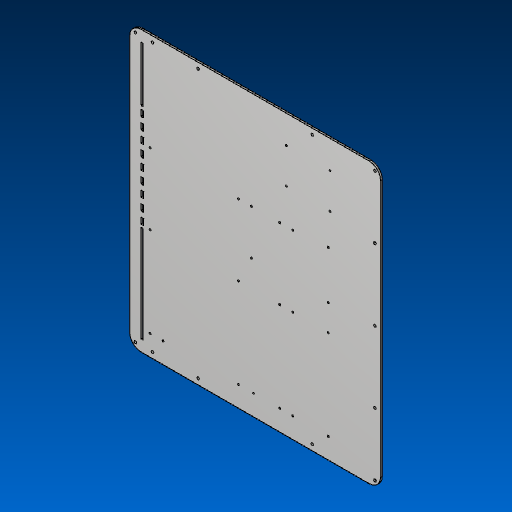
# Autodesk Inventor part: right_panel
Saved by Autodesk Inventor 2018 (Build 220112000, 112)
## iProperties
Created: 2019-10-14
Part Number: right_panel
Material: アルミニウム 6061
Document SubType Name: Modeling
Designer: gisen
Density: 2.7 g/cm^3
Appearance: アルミニウム - フラット
Author: gisen
Autodesk Inventor part; units mm, degrees
ref_plane "YZ Plane" through (0, 0, 0) normal (1, 0, 0) x (0, 1, 0)
ref_plane "XZ Plane" through (0, 0, 0) normal (0, 1, 0) x (-1, 0, 0)
ref_plane "XY Plane" through (0, 0, 0) normal (0, 0, 1) x (1, 0, 0)
sketch "スケッチ1" plane through (0, 0, 0) normal (0, 0, 1) x (1, 0, 0)
  line L0 (-200, -245) -> (200, -245)
  line L1 (220, -225) -> (220, 225)
  line L2 (200, 245) -> (-200, 245)
  line L3 (-220, 225) -> (-220, -225)
  line L4 (-220, -245) -> (220, 245) construction
  line L5 (220, -245) -> (-220, 245) construction
  circle A0 centre (-210, 235) radius 2.25
  circle A1 centre (210, 235) radius 2.25
  circle A2 centre (-210, -235) radius 2.25
  circle A3 centre (210, -235) radius 2.25
  arc A4 (-200, 245) -> (-220, 225) centre (-200, 225) ccw
  arc A5 (220, 225) -> (200, 245) centre (200, 225) ccw
  arc A6 (200, -245) -> (220, -225) centre (200, -225) ccw
  arc A7 (-220, -225) -> (-200, -245) centre (-200, -225) ccw
  point P0 (0, 0)
  dimension "d0" = 440
  dimension "d1" = 490
  dimension "d2" = 4.5
  dimension "d3" = 10
  dimension "d4" = 10
  dimension "d5" = 10
  dimension "d6" = 10
  dimension "d7" = 10
  dimension "d8" = 10
  dimension "d9" = 10
  dimension "d10" = 10
  dimension "d11" = 20
  constraints: 12 end point, 8 centre point, 8 point on circle, 8 point on line, 8 tangent, 6 equal radius, 2 midpoint, 2 parallel, 1 horizontal, 1 perpendicular
  measures "d0" distance of L5.end L4.end
  measures "d1" distance of L4.end L5.start
  measures "d2" diameter of A0
  measures "d3" distance from line of A0.centre L2
  measures "d4" distance from line of L3 A0.centre
  measures "d5" distance from line of A1.centre L2
  measures "d6" distance from line of L1 A1.centre
  measures "d7" distance from line of L1 A3.centre
  measures "d8" distance from line of L0 A3.centre
  measures "d9" distance from line of L0 A2.centre
  measures "d10" distance from line of L3 A2.centre
  measures "d11" radius of A4
extrude "押し出し1" add sketch "スケッチ1" along normal blind 3
sketch "スケッチ2" plane through (0, 0, 3) normal (0, 0, 1) x (1, 0, 0)
  circle A0 centre (43.092, 72.9258) radius 1.6
  circle A1 centre (-29.298, 72.9258) radius 1.6
  circle A2 centre (-184.238, 72.9258) radius 1.6
  circle A3 centre (-184.238, -51.5342) radius 1.6
  circle A4 centre (-161.378, -209.0142) radius 1.6
  circle A5 centre (-29.298, -209.0142) radius 1.6
  circle A6 centre (43.092, -209.0142) radius 1.6
  circle A7 centre (43.092, -51.5342) radius 1.6
  circle A8 centre (-29.298, -51.5342) radius 1.6
  circle A9 centre (43.092, -209.0142) radius 2.25 projected
  circle A10 centre (-161.378, -209.0142) radius 2.25 projected
  circle A11 centre (43.092, -51.5342) radius 2.25 projected
  circle A12 centre (43.092, 72.9258) radius 2.25 projected
  circle A13 centre (-29.298, -209.0142) radius 2.25 projected
  circle A14 centre (-29.298, -51.5342) radius 2.25 projected
  circle A15 centre (-29.298, 72.9258) radius 2.25 projected
  circle A16 centre (-184.238, -51.5342) radius 2.25 projected
  circle A17 centre (-184.238, 72.9258) radius 2.25 projected
  point P0 (0, 0)
  dimension "d14" = 3.2
  constraints: 9 centre point, 9 concentric, 8 equal radius
  measures "d14" diameter of A0
extrude "押し出し2" cut sketch "スケッチ2" against normal blind 3 contours A0 | A1 | A2 | A3 | A4 | A5 | A6 | A7 | A8
sketch "スケッチ4" plane through (0, 0, 3) normal (0, 0, 1) x (1, 0, 0)
  line L0 (-200, -225) -> (-197, -225) projected
  line L1 (-200, -30.5483) -> (-200, -20.2613) projected
  line L2 (-200, -30.5483) -> (-197, -30.5483) projected
  line L3 (-197, -20.2613) -> (-197, -30.5483) projected
  line L4 (-200, -20.2613) -> (-197, -20.2613) projected
  line L5 (-200, -9.8937) -> (-200, 0.3933) projected
  line L6 (-200, -9.8937) -> (-197, -9.8937) projected
  line L7 (-197, 0.3933) -> (-197, -9.8937) projected
  line L8 (-200, 0.3933) -> (-197, 0.3933) projected
  line L9 (-200, 10.4517) -> (-200, 20.7387) projected
  line L10 (-200, 10.4517) -> (-197, 10.4517) projected
  line L11 (-197, 20.7387) -> (-197, 10.4517) projected
  line L12 (-200, 20.7387) -> (-197, 20.7387) projected
  line L13 (-200, 31.1063) -> (-200, 41.3933) projected
  line L14 (-200, 31.1063) -> (-197, 31.1063) projected
  line L15 (-197, 41.3933) -> (-197, 31.1063) projected
  line L16 (-200, 41.3933) -> (-197, 41.3933) projected
  line L17 (-200, 51.4517) -> (-200, 61.7387) projected
  line L18 (-200, 51.4517) -> (-197, 51.4517) projected
  line L19 (-197, 61.7387) -> (-197, 51.4517) projected
  line L20 (-200, 61.7387) -> (-197, 61.7387) projected
  line L21 (-200, 72.1063) -> (-200, 82.3933) projected
  line L22 (-200, 72.1063) -> (-197, 72.1063) projected
  line L23 (-197, 82.3933) -> (-197, 72.1063) projected
  line L24 (-200, 82.3933) -> (-197, 82.3933) projected
  line L25 (-200, 92.4517) -> (-200, 102.7387) projected
  line L26 (-200, 92.4517) -> (-197, 92.4517) projected
  line L27 (-197, 102.7387) -> (-197, 92.4517) projected
  line L28 (-200, 102.7387) -> (-197, 102.7387) projected
  line L29 (-200, 225) -> (-200, 129.6) projected
  line L30 (-200, 129.6) -> (-197, 129.6) projected
  line L31 (-197, 225) -> (-197, 129.6) projected
  line L32 (-200, 225) -> (-197, 225) projected
  line L33 (-197, 102.7387) -> (-196, 102.7387)
  line L34 (-196, 102.7387) -> (-196, 92.4517)
  line L35 (-196, 92.4517) -> (-197, 92.4517)
  line L36 (-197, 82.3933) -> (-196, 82.3933)
  line L37 (-196, 82.3933) -> (-196, 72.1063)
  line L38 (-196, 72.1063) -> (-197, 72.1063)
  line L39 (-197, 61.7387) -> (-196, 61.7387)
  line L40 (-196, 61.7387) -> (-196, 51.4517)
  line L41 (-196, 51.4517) -> (-197, 51.4517)
  line L42 (-197, 41.3933) -> (-196, 41.3933)
  line L43 (-196, 41.3933) -> (-196, 31.1063)
  line L44 (-196, 31.1063) -> (-197, 31.1063)
  line L45 (-197, 20.7387) -> (-196, 20.7387)
  line L46 (-196, 20.7387) -> (-196, 10.4517)
  line L47 (-196, 10.4517) -> (-197, 10.4517)
  line L48 (-197, 0.3933) -> (-196, 0.3933)
  line L49 (-196, 0.3933) -> (-196, -9.8937)
  line L50 (-196, -9.8937) -> (-197, -9.8937)
  line L51 (-197, -20.2613) -> (-196, -20.2613)
  line L52 (-196, -20.2613) -> (-196, -30.5483)
  line L53 (-196, -30.5483) -> (-197, -30.5483)
  line L54 (-197, -40.6067) -> (-196, -40.6067)
  line L55 (-196, -40.6067) -> (-196, -50.8937)
  line L56 (-196, -50.8937) -> (-197, -50.8937)
  line L57 (-200, -225) -> (-200, -56.0642) projected
  line L58 (-197, -56.0642) -> (-197, -225) projected
  line L59 (-200, 112.7971) -> (-197, 112.7971) projected
  line L60 (-200, 123.0841) -> (-200, 112.7971) projected
  line L61 (-200, 123.0841) -> (-197, 123.0841) projected
  line L62 (-197, 112.7971) -> (-196, 112.7971)
  line L63 (-196, 112.7971) -> (-196, 123.0841)
  line L64 (-196, 123.0841) -> (-197, 123.0841)
  line L65 (-197, -40.6067) -> (-197, -50.8937) construction
  line L66 (-197, -50.8937) -> (-200, -50.8937)
  line L67 (-200, -50.8937) -> (-200, -40.6067)
  line L68 (-200, -40.6067) -> (-197, -40.6067)
  line L69 (-200, -56.0642) -> (-197, -56.0642) projected
  point P0 (0, 0)
  point P1 (-225, -58.3552)
  point P2 (-222, -58.3552)
  point P3 (-225, -120.4005)
  point P4 (-222, -120.4005)
  dimension "d17" = 1
  constraints: 60 end point, 17 perpendicular, 10 equal length, 10 horizontal, 2 collinear, 4 other
  measures "d17" distance of L27.start L33.end
extrude "押し出し3" cut sketch "スケッチ4" against normal blind 3
sketch "スケッチ5" plane through (0, 0, 3) normal (0, 0, 1) x (1, 0, 0)
  circle A0 centre (-210, 235) radius 2.25 construction
  circle A1 centre (-210, -235) radius 2.25 construction
  circle A2 centre (-180, -235) radius 2.25
  line L0 (-200, -245) -> (200, -245) projected
  circle A3 centre (-180, 235) radius 2.25
  line L1 (200, 245) -> (-200, 245) projected
  point P0 (0, 0)
  dimension "d20" = 30
  dimension "d21" = 10
  dimension "d22" = 30
  dimension "d23" = 10
  constraints: 2 centre point, 2 equal radius
  measures "d20" distance of A1.centre A2.centre
  measures "d21" distance from line of L0 A2.centre
  measures "d22" distance of A0.centre A3.centre
  measures "d23" distance from line of L1 A3.centre
extrude "押し出し4" cut sketch "スケッチ5" against normal blind 3
sketch "スケッチ6" plane through (0, 0, 3) normal (0, 0, 1) x (1, 0, 0)
  circle A0 centre (-180, -235) radius 2.25 construction
  circle A1 centre (-180, 235) radius 2.25 construction
  circle A2 centre (43.092, -51.5342) radius 1.6 construction
  circle A3 centre (-29.298, -209.0142) radius 1.6 construction
  circle A4 centre (-184.238, -51.5342) radius 1.6 construction
  circle A5 centre (-29.298, 72.9258) radius 1.6 construction
  circle A6 centre (43.092, 72.9258) radius 1.6 construction
  circle A7 centre (-184.238, 72.9258) radius 1.6 construction
  circle A8 centre (-161.378, -209.0142) radius 1.6 construction
  circle A9 centre (43.092, -209.0142) radius 1.6 construction
  circle A10 centre (-29.298, -51.5342) radius 1.6 construction
  circle A11 centre (210, -235) radius 2.25 construction
  circle A12 centre (-210, -235) radius 2.25 construction
  circle A13 centre (210, 235) radius 2.25 construction
  circle A14 centre (-210, 235) radius 2.25 construction
  line L0 (200, 245) -> (-200, 245) construction
  arc A15 (-200, 245) -> (-220, 225) centre (-200, 225) ccw construction
  arc A16 (-220, -225) -> (-200, -245) centre (-200, -225) ccw construction
  line L1 (-200, -245) -> (200, -245) construction
  arc A17 (200, -245) -> (220, -225) centre (200, -225) ccw construction
  line L2 (220, -225) -> (220, 225) construction
  arc A18 (220, 225) -> (200, 245) centre (200, 225) ccw construction
  line L3 (-196.8, 129.4) -> (-200.2, 129.4)
  line L4 (-200.2, 129.4) -> (-200.2, 225.2)
  line L5 (-200.2, 225.2) -> (-196.8, 225.2)
  line L6 (-196.8, 225.2) -> (-196.8, 129.4)
  line L7 (-195.8, 102.9387) -> (-195.8, 92.2517)
  line L8 (-195.8, 92.2517) -> (-200.2, 92.2517)
  line L9 (-200.2, 92.2517) -> (-200.2, 102.9387)
  line L10 (-200.2, 102.9387) -> (-195.8, 102.9387)
  line L11 (-195.8, 82.5933) -> (-195.8, 71.9063)
  line L12 (-195.8, 71.9063) -> (-200.2, 71.9063)
  line L13 (-200.2, 71.9063) -> (-200.2, 82.5933)
  line L14 (-200.2, 82.5933) -> (-195.8, 82.5933)
  line L15 (-195.8, 61.9387) -> (-195.8, 51.2517)
  line L16 (-195.8, 51.2517) -> (-200.2, 51.2517)
  line L17 (-200.2, 51.2517) -> (-200.2, 61.9387)
  line L18 (-200.2, 61.9387) -> (-195.8, 61.9387)
  line L19 (-195.8, 41.5933) -> (-195.8, 30.9063)
  line L20 (-195.8, 30.9063) -> (-200.2, 30.9063)
  line L21 (-200.2, 30.9063) -> (-200.2, 41.5933)
  line L22 (-200.2, 41.5933) -> (-195.8, 41.5933)
  line L23 (-195.8, 20.9387) -> (-195.8, 10.2517)
  line L24 (-195.8, 10.2517) -> (-200.2, 10.2517)
  line L25 (-200.2, 10.2517) -> (-200.2, 20.9387)
  line L26 (-200.2, 20.9387) -> (-195.8, 20.9387)
  line L27 (-195.8, 0.5933) -> (-195.8, -10.0937)
  line L28 (-195.8, -10.0937) -> (-200.2, -10.0937)
  line L29 (-200.2, -10.0937) -> (-200.2, 0.5933)
  line L30 (-200.2, 0.5933) -> (-195.8, 0.5933)
  line L31 (-195.8, -20.0613) -> (-195.8, -30.7483)
  line L32 (-195.8, -30.7483) -> (-200.2, -30.7483)
  line L33 (-200.2, -30.7483) -> (-200.2, -20.0613)
  line L34 (-200.2, -20.0613) -> (-195.8, -20.0613)
  line L35 (-195.8, -40.4067) -> (-195.8, -51.0937)
  line L36 (-195.8, -51.0937) -> (-200.2, -51.0937)
  line L37 (-200.2, -51.0937) -> (-200.2, -40.4067)
  line L38 (-200.2, -40.4067) -> (-195.8, -40.4067)
  line L39 (-196.8, -55.8642) -> (-200.2, -55.8642)
  line L40 (-200.2, -55.8642) -> (-200.2, -225.2)
  line L41 (-200.2, -225.2) -> (-196.8, -225.2)
  line L42 (-196.8, -225.2) -> (-196.8, -55.8642)
  line L43 (-196, -50.8937) -> (-200, -50.8937) projected
  line L44 (-200, -40.6067) -> (-196, -40.6067) projected
  line L45 (-195.8, 112.5971) -> (-200.2, 112.5971)
  line L46 (-200.2, 112.5971) -> (-200.2, 123.2841)
  line L47 (-200.2, 123.2841) -> (-195.8, 123.2841)
  line L48 (-195.8, 123.2841) -> (-195.8, 112.5971)
  line L49 (-196, 112.7971) -> (-200, 112.7971) projected
  line L50 (-200, 123.0841) -> (-196, 123.0841) projected
  line L51 (-220, 225) -> (-220, -225) projected
  line L52 (-197, 129.6) -> (-200, 129.6) projected
  line L53 (-200, 123.0841) -> (-196, 123.0841) projected
  line L54 (-196, 123.0841) -> (-196, 112.7971) projected
  line L55 (-196, 112.7971) -> (-200, 112.7971) projected
  line L56 (-200, 102.7387) -> (-196, 102.7387) projected
  line L57 (-196, 102.7387) -> (-196, 92.4517) projected
  line L58 (-196, 92.4517) -> (-200, 92.4517) projected
  line L59 (-200, 82.3933) -> (-196, 82.3933) projected
  line L60 (-196, 82.3933) -> (-196, 72.1063) projected
  line L61 (-196, 72.1063) -> (-200, 72.1063) projected
  line L62 (-200, 61.7387) -> (-196, 61.7387) projected
  line L63 (-196, 61.7387) -> (-196, 51.4517) projected
  line L64 (-196, 51.4517) -> (-200, 51.4517) projected
  line L65 (-200, 41.3933) -> (-196, 41.3933) projected
  line L66 (-196, 41.3933) -> (-196, 31.1063) projected
  line L67 (-196, 31.1063) -> (-200, 31.1063) projected
  line L68 (-200, 20.7387) -> (-196, 20.7387) projected
  line L69 (-196, 20.7387) -> (-196, 10.4517) projected
  line L70 (-196, 10.4517) -> (-200, 10.4517) projected
  line L71 (-200, 0.3933) -> (-196, 0.3933) projected
  line L72 (-196, 0.3933) -> (-196, -9.8937) projected
  line L73 (-196, -9.8937) -> (-200, -9.8937) projected
  line L74 (-200, -20.2613) -> (-196, -20.2613) projected
  line L75 (-196, -20.2613) -> (-196, -30.5483) projected
  line L76 (-196, -30.5483) -> (-200, -30.5483) projected
  line L77 (-197, -56.0642) -> (-197, -225) projected
  line L78 (-197, -225) -> (-200, -225) projected
  line L79 (-200, 225) -> (-197, 225) projected
  line L80 (-197, 225) -> (-197, 129.6) projected
  line L81 (-200, 129.6) -> (-200, 225) projected
  line L82 (-200, 92.4517) -> (-200, 102.7387) projected
  line L83 (-200, 51.4517) -> (-200, 61.7387) projected
  line L84 (-200, 10.4517) -> (-200, 20.7387) projected
  line L85 (-200, -9.8937) -> (-200, 0.3933) projected
  line L86 (-200, -30.5483) -> (-200, -20.2613) projected
  line L87 (-200, 31.1063) -> (-200, 41.3933) projected
  line L88 (-200, 72.1063) -> (-200, 82.3933) projected
  line L89 (-200, 112.7971) -> (-200, 123.0841) projected
  line L90 (-200, -40.6067) -> (-196, -40.6067) projected
  line L91 (-196, -40.6067) -> (-196, -50.8937) projected
  line L92 (-196, -50.8937) -> (-200, -50.8937) projected
  line L93 (-200, -56.0642) -> (-197, -56.0642) projected
  line L94 (-200, -50.8937) -> (-200, -40.6067) projected
  line L95 (-200, -225) -> (-200, -56.0642) projected
  point P0 (0, 0)
  point P1 (-197, -40.6067)
  point P2 (-197, -50.8937)
  dimension "d81" = 0.2
  dimension "d82" = 0.2
  dimension "d97" = 0.2
  dimension "d98" = 0.2
  dimension "d101" = 0.2
  dimension "d106" = 0.2
  dimension "d107" = 0.2
  dimension "d108" = 0.2
  dimension "d109" = 0.2
  dimension "d110" = 0.2
  dimension "d111" = 0.2
  dimension "d112" = 0.2
  dimension "d113" = 0.2
  dimension "d114" = 0.2
  dimension "d115" = 0.2
  dimension "d116" = 0.2
  dimension "d117" = 0.2
  dimension "d118" = 0.2
  dimension "d119" = 0.2
  dimension "d120" = 0.2
  dimension "d121" = 0.2
  dimension "d122" = 0.2
  dimension "d123" = 0.2
  dimension "d124" = 0.2
  dimension "d127" = 0.2
  constraints: 88 end point, 17 vertical, 17 vertical alignment, 4 point on circle, 3 horizontal, 2 centre point, 2 parallel, 2 perpendicular
  measures "d81" distance between parallel lines of L36 L43
  measures "d82" distance between parallel lines of L38 L44
  measures "d97" distance between parallel lines of L49 L45
  measures "d98" distance between parallel lines of L47 L50
  measures "d101" distance from line of L35 L43.start
  measures "d106" distance from line of L5.end L80
  measures "d107" distance between parallel lines of L81 L4
  measures "d108" distance between parallel lines of L79 L5
  measures "d109" distance between parallel lines of L3 L52
  measures "d110" distance between parallel lines of L56 L10
  measures "d111" distance between parallel lines of L8 L58
  measures "d112" distance between parallel lines of L14 L59
  measures "d113" distance between parallel lines of L12 L61
  measures "d114" distance between parallel lines of L62 L18
  measures "d115" distance between parallel lines of L16 L64
  measures "d116" distance between parallel lines of L65 L22
  measures "d117" distance between parallel lines of L67 L20
  measures "d118" distance between parallel lines of L26 L68
  measures "d119" distance between parallel lines of L24 L70
  measures "d120" distance between parallel lines of L71 L30
  measures "d121" distance between parallel lines of L28 L73
  measures "d122" distance between parallel lines of L74 L34
  measures "d123" distance between parallel lines of L32 L76
  measures "d124" distance between parallel lines of L42 L77
  measures "d127" distance between parallel lines of L41 L78
extrude "押し出し5" cut sketch "スケッチ6" against normal through all contours L3 L4 L5 L6 | L7 L8 L9 L10 | L11 L12 L13 L14 | L15 L16 L17 L18 | L19 L20 L21 L22 | L23 L24 L25 L26 | L27 L28 L29 L30 | L31 L32 L33 L34 | L35 L36 L37 L38 | L42 L41 L40 L39 | L43 L94 L44 L91 | L45 L46 L47 L48 | L49 L89 L50 L54 | L52 L81 L79 L80 | L56 L57 L58 L82 | L59 L60 L61 L88 | L62 L63 L64 L83 | L65 L66 L67 L87 | L68 L69 L70 L84 | L71 L72 L73 L85 | L74 L75 L76 L86 | L77 L78 L95 L93
sketch "スケッチ7" plane through (0, 0, 3) normal (0, 0, 1) x (1, 0, 0)
  line L0 (220, 225) -> (220, -225) projected
  circle A0 centre (-100, -235) radius 2.25 projected
  circle A1 centre (210, 0) radius 2.25 projected
  circle A2 centre (100, -235) radius 2.25 projected
  circle A3 centre (210, 125) radius 2.25 projected
  circle A4 centre (-100, 235) radius 2.25 projected
  circle A5 centre (-210, -125) radius 2.25 projected
  circle A6 centre (-210, 0) radius 2.25 projected
  circle A7 centre (100, 235) radius 2.25 projected
  circle A8 centre (210, -125) radius 2.25 projected
  line L1 (-200.2, 132.4) -> (-196.8, 132.4) projected
  line L2 (-196.8, 132.4) -> (-196.8, 225.2) projected
  line L3 (-196.8, 225.2) -> (-200.2, 225.2) projected
  circle A9 centre (210, 235) radius 2.25 projected
  circle A10 centre (-210, 235) radius 2.25 projected
  circle A11 centre (210, -235) radius 2.25 projected
  circle A12 centre (-210, -235) radius 2.25 projected
  line L4 (200, -245) -> (-200, -245) projected
  arc A13 (-220, -225) -> (-200, -245) centre (-200, -225) ccw projected
  line L5 (-220, -225) -> (-220, 225) projected
  arc A14 (-200, 245) -> (-220, 225) centre (-200, 225) ccw projected
  line L6 (-200, 245) -> (200, 245) projected
  arc A15 (220, 225) -> (200, 245) centre (200, 225) ccw projected
  line L7 (220, 225) -> (220, -225) projected
  arc A16 (200, -245) -> (220, -225) centre (200, -225) ccw projected
  circle A17 centre (-210, 125) radius 2.25 projected
  line L8 (-200.2, 225.2) -> (-200.2, 132.4) projected
  point P0 (0, 0)
  point P1 (-212.7501, 124.9816)
  point P2 (-217.2499, 124.9816)
  constraints: 1 other
extrude "押し出し6" cut sketch "スケッチ7" against normal up to surface (3 mm away) contours A0 | A1 | A2 | A3 | A4 | A7 | A8
sketch "スケッチ8" plane through (0, 0, 0) normal (0, 0, -1) x (-1, 0, 0)
  line L0 (-44.775, 130.075) -> (-145.225, 130.075) construction
  line L1 (-145.225, 130.075) -> (-145.225, 199.925) construction
  line L2 (-145.225, 199.925) -> (-44.775, 199.925) construction
  line L3 (-44.775, 199.925) -> (-44.775, 130.075) construction
  line L4 (-44.775, 130.075) -> (-145.225, 199.925) construction
  line L5 (-145.225, 130.075) -> (-44.775, 199.925) construction
  line L6 (200, 245) -> (-200, 245) construction
  line L7 (-220, 225) -> (-220, -225) construction
  line L8 (-54.625, 195.86) -> (-131.225, 195.86) construction
  line L9 (-131.225, 195.86) -> (-131.225, 134.14) construction
  line L10 (-131.225, 134.14) -> (-54.625, 134.14) construction
  line L11 (-54.625, 134.14) -> (-54.625, 195.86) construction
  line L12 (-54.625, 195.86) -> (-131.225, 134.14) construction
  line L13 (-131.225, 195.86) -> (-54.625, 134.14) construction
  line L14 (-92.925, 165) -> (-95, 165) construction
  circle A0 centre (-54.625, 134.14) radius 1.6
  circle A1 centre (-54.625, 195.86) radius 1.6
  circle A2 centre (-131.225, 195.86) radius 1.6
  circle A3 centre (-131.225, 134.14) radius 1.6
  point P0 (0, 0)
  dimension "d40" = 69.85
  dimension "d41" = 100.45
  dimension "d42" = 80
  dimension "d43" = 125
  dimension "d44" = 61.72
  dimension "d45" = 90.6
  dimension "d46" = 14
  dimension "d47" = 3.2
  dimension "d48" = 3.2
  dimension "d49" = 3.2
  dimension "d50" = 3.2
  constraints: 26 end point, 4 centre point, 4 coincident, 4 midpoint, 4 parallel, 3 horizontal, 2 perpendicular
  measures "d40" distance of L0.end L1.end
  measures "d41" distance of L0.start L0.end
  measures "d42" distance from line of L6 L14.end
  measures "d43" distance from line of L7 L14.end
  measures "d44" distance of L10.end L8.start
  measures "d45" distance between parallel lines of L1 L11
  measures "d46" distance between parallel lines of L1 L9
  measures "d47" diameter of A0
  measures "d48" diameter of A1
  measures "d49" diameter of A2
  measures "d50" diameter of A3
extrude "押し出し7" cut sketch "スケッチ8" against normal through all
sketch "スケッチ9" plane through (0, 0, 0) normal (0, 0, -1) x (-1, 0, 0)
  circle A0 centre (161.378, -209.0142) radius 1.6 construction
  circle A1 centre (29.298, -209.0142) radius 1.6 construction
  circle A2 centre (-43.092, -209.0142) radius 1.6 construction
  circle A3 centre (184.238, -51.5342) radius 1.6 construction
  circle A4 centre (184.238, 72.9258) radius 1.6 construction
  circle A5 centre (29.298, 72.9258) radius 1.6 construction
  circle A6 centre (-43.092, 72.9258) radius 1.6 construction
  circle A7 centre (29.298, -51.5342) radius 1.6 construction
  circle A8 centre (-43.092, -51.5342) radius 1.6 construction
  line L0 (194.398, -215.3642) -> (-77.382, -215.3642) construction
  line L1 (-77.382, -215.3642) -> (-77.382, 89.4358) construction
  line L2 (-77.382, 89.4358) -> (194.398, 89.4358) construction
  line L3 (194.398, 89.4358) -> (194.398, -215.3642) construction
  point P0 (0, 0)
  dimension "d53" = 6.35
  dimension "d54" = 33.02
  dimension "d55" = 304.8
  dimension "d56" = 271.78
  constraints: 8 end point, 2 parallel, 1 horizontal, 1 perpendicular
  measures "d53" distance from line of A0.centre L0
  measures "d54" distance from line of L3 A0.centre
  measures "d55" distance of L2.end L0.start
  measures "d56" distance of L0.start L0.end
sketch "スケッチ10" plane through (0, 0, 0) normal (0, 0, -1) x (-1, 0, 0)
  line L0 (194.398, -215.3642) -> (-135.802, -215.3642) construction
  line L1 (-135.802, -215.3642) -> (-135.802, 89.4358) construction
  line L2 (-135.802, 89.4358) -> (194.398, 89.4358) construction
  line L3 (194.398, 89.4358) -> (194.398, -215.3642) construction
  circle A0 centre (184.238, 72.9258) radius 1.6 construction
  circle A1 centre (-210, -125) radius 2.25 projected
  circle A2 centre (-128.182, 78.0058) radius 1.6
  circle A3 centre (184.238, 72.9258) radius 1.6 construction
  line L4 (184.238, 72.9258) -> (29.298, 72.9258) construction
  circle A4 centre (29.298, 72.9258) radius 1.6 construction
  circle A5 centre (29.298, 72.9258) radius 1.6 construction
  line L5 (29.298, 72.9258) -> (-43.092, 72.9258) construction
  line L6 (-43.092, 72.9258) -> (-65.952, 72.9258) construction
  circle A6 centre (-43.092, 72.9258) radius 1.6
  circle A7 centre (-65.952, 72.9258) radius 1.6
  line L7 (-128.182, 78.0058) -> (-128.182, -5.8142) construction
  line L8 (-128.182, -5.8142) -> (-128.182, -51.5342) construction
  line L9 (-128.182, -51.5342) -> (-128.182, -208.9142) construction
  circle A8 centre (-128.182, -5.8142) radius 1.6
  circle A9 centre (-128.182, -51.5342) radius 1.6
  circle A10 centre (-128.182, -208.9142) radius 1.6
  line L10 (-128.182, -5.8142) -> (6.438, -5.8142) construction
  circle A11 centre (6.438, -5.8142) radius 1.6
  line L11 (6.438, -5.8142) -> (6.438, 72.9258) construction
  circle A12 centre (6.438, 72.9258) radius 1.6
  line L12 (184.238, 72.9258) -> (184.238, -209.0142) construction
  circle A13 centre (161.378, -209.0142) radius 1.6 construction
  line L13 (184.238, -209.0142) -> (161.378, -209.0142) construction
  circle A14 centre (184.238, -209.0142) radius 1.6
  line L14 (-65.952, 72.9258) -> (-65.952, -209.0142) construction
  line L15 (-65.952, -209.0142) -> (-43.092, -209.0142) construction
  circle A15 centre (-43.092, -51.5342) radius 1.6 construction
  line L16 (-43.092, -51.5342) -> (-65.952, -51.5342) construction
  circle A16 centre (-43.092, -209.0142) radius 1.6 construction
  circle A17 centre (-65.952, -51.5342) radius 1.6
  circle A18 centre (-65.952, -209.0142) radius 1.6
  line L17 (-43.092, -209.0142) -> (161.378, -209.0142) construction
  circle A19 centre (2.628, -209.0142) radius 1.6
  point P0 (0, 0)
  dimension "d57" = 330.2
  dimension "d58" = 304.8
  dimension "d59" = 10.16
  dimension "d60" = 16.51
  dimension "d61" = 74.198
  dimension "d62" = 5.08
  dimension "d63" = 312.42
  dimension "d64" = 154.94
  dimension "d65" = 227.33
  dimension "d66" = 250.19
  dimension "d67" = 78.74
  dimension "d68" = 124.46
  dimension "d69" = 281.84
  dimension "d70" = 177.8
  dimension "d71" = 134.62
  dimension "d72" = 16.51
  dimension "d73" = 181.61
  dimension "d74" = 3.2
  constraints: 36 end point, 14 centre point, 13 coincident, 13 equal radius, 6 point on line, 5 horizontal, 4 perpendicular, 4 vertical, 2 parallel
  measures "d57" distance of L0.start L0.end
  measures "d58" distance of L0.end L1.end
  measures "d59" distance from line of A0.centre L3
  measures "d60" distance from line of L2 A0.centre
  measures "d61" distance from line of L1 A1.centre
  measures "d62" vertical distance of A0.centre L7.start
  measures "d63" horizontal distance of A0.centre L7.start
  measures "d64" distance of L4.start L4.end
  measures "d65" distance of L5.end L4.start
  measures "d66" distance of L4.start L6.end
  measures "d67" vertical distance of L10.start A0.centre
  measures "d68" vertical distance of L8.end A0.centre
  measures "d69" vertical distance of L4.start L9.end
  measures "d70" horizontal distance of L4.start L10.end
  measures "d71" distance of L10.start L10.end
  measures "d72" distance from line of L2 L11.end
  measures "d73" distance from line of L12 A19.centre
  measures "d74" diameter of A0
extrude "押し出し8" cut sketch "スケッチ10" against normal blind 10 contours A2 | A7 | A8 | A9 | A10 | A11 | A12 | A14 | A17 | A18 | A19
equation "\"d5\" = d3"
equation "\"d6\" = d4"
equation "\"d7\" = d6"
equation "\"d8\" = d5"
equation "\"d9\" = d8"
equation "\"d10\" = d7"
